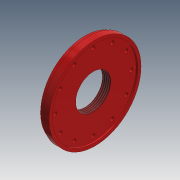
# Autodesk Inventor part: P302Base
Saved by Autodesk Inventor 2017 (Build 210142000, 142)
## iProperties
Created: 2017-11-15
Part Number: P302Base
Material: ABS Plastic
Document SubType Name: Modeling
Designer: serge.amoos
Density: 1.06 g/cm^3
Appearance: Light Red
Author: serge.amoos
Autodesk Inventor part; units mm, degrees
ref_plane "YZ Plane" through (0, 0, 0) normal (1, 0, 0) x (0, 1, 0)
ref_plane "XZ Plane" through (0, 0, 0) normal (0, 1, 0) x (-1, 0, 0)
ref_plane "XY Plane" through (0, 0, 0) normal (0, 0, 1) x (1, 0, 0)
sketch "Sketch1" plane through (0, 0, 0) normal (0, 0, 1) x (1, 0, 0)
  line L0 (-6.6, 0) -> (1.1, 0) construction
  line L1 (0, -4.95) -> (0, 29.7) construction
  line L2 (-1, 9.5) -> (-1, 23.1)
  line L3 (-1, 23.1) -> (0, 23.1)
  line L4 (0, 23.1) -> (0, 24.75)
  line L5 (0, 24.75) -> (-3.5, 24.75)
  line L6 (-3.5, 24.75) -> (-3.5, 23.9)
  line L7 (-3.5, 23.9) -> (-5.5, 23.9)
  line L8 (-5.5, 23.9) -> (-5.5, 9.5)
  line L9 (-5.5, 9.5) -> (-1, 9.5)
  point P0 (0, 0)
  dimension "d0" = 49.5
  dimension "d1" = 47.8
  dimension "d2" = 19
  dimension "d3" = 2
  dimension "d4" = 1
  dimension "d5" = 5.5
  dimension "d6" = 46.2
  constraints: 16 end point, 5 perpendicular, 2 point on line, 1 horizontal, 1 vertical
  measures "d0" diameter of L5 L0
  measures "d1" diameter of L7 L0
  measures "d2" diameter of L9 L0
  measures "d3" distance of L6.end L7.end
  measures "d4" distance of L2.end L3.end
  measures "d5" distance between parallel lines of L4 L8
  measures "d6" diameter of L3 L0
revolve "Revolution1" add sketch "Sketch1" angle 360 about axis through (-10, 0, 0) along (1, 0, 0)
sketch "Sketch2" plane through (-1, 0, 0) normal (1, 0, 0) x (0, 0, -1)
  line L0 (0, -34.65) -> (0, 34.65) projected
  line L1 (34.65, 0) -> (-34.65, 0) projected
  point P0 (0, 0)
  point P1 (-20.5, 0)
  dimension "d8" = 20.5
  constraints: 1 point on line
  measures "d8" distance from line of L0 point (-20.5, 0)
hole "Hole1" at (-1, 0, 20.5) direction (-1, 0, 0) diameter 2 end through all
pattern_circular "Circular Pattern1" count 12 over 360 about axis through (-10, 0, 0) along (1, 0, 0) of "Hole1"
thread "Thread1" size "M20x1" class "6H" standard "ISO Metric profile" full length
body "Solid1"
